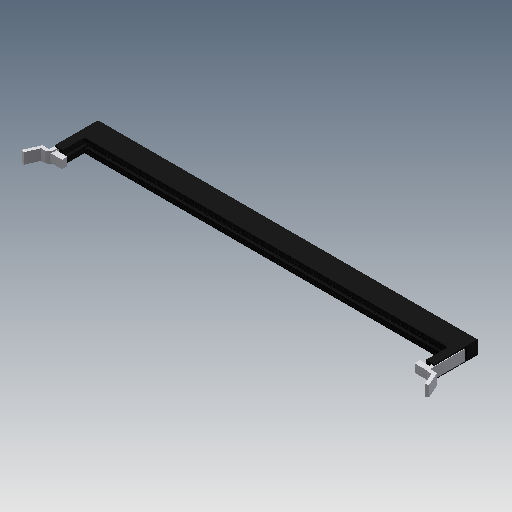
# Autodesk Inventor part: config - ram slot
Saved by Autodesk Inventor 2019.1 (Build 231200000, 200)
## iProperties
Company: Autodesk Asia Pte. Ltd.
Created: 2005-11-27
Part Number: config - ram slot
Document SubType Name: Modeling
Designer: Simon.Ng@autodesk.com
Stock Number: config - ram slot
Density: 1 g/cm^3
Material: Generic
Mass: 5.26159 g
Surface Area: 74.6749 cm^2
Volume: 5.26159 cm^3
Appearance: Glossy - Black
Title: PC Demo
Author: Simon.Ng@autodesk.com
Autodesk Inventor part; units mm, degrees
ref_plane "YZ Plane" through (0, 0, 0) normal (1, 0, 0) x (0, 1, 0)
ref_plane "XZ Plane" through (0, 0, 0) normal (0, 1, 0) x (-1, 0, 0)
ref_plane "XY Plane" through (0, 0, 0) normal (0, 0, 1) x (1, 0, 0)
sketch "Sketch1" plane through (0, 0, 0) normal (0, 0, 1) x (1, 0, 0)
  line L0 (0, 6.5) -> (0, -0.5) projected
  line L1 (-14, 0) -> (182, 0) projected
  line L2 (0, 0) -> (140, 0)
  line L3 (140, 0) -> (140, 5)
  line L4 (140, 5) -> (0, 5)
  line L5 (0, 5) -> (0, 0)
  dimension "d0" = 140
  dimension "d1" = 5
  constraints: 8 end point, 2 parallel, 2 point on line, 1 horizontal, 1 perpendicular
  measures "d0" distance of L3.end L4.end
  measures "d1" distance of L2.end L3.end
extrude "Extrusion1" add sketch "Sketch1" along normal blind 16
sketch "Sketch2" plane through (0, 0, 16) normal (0, 0, 1) x (1, 0, 0)
  line L0 (0, 0) -> (0, 5) projected
  line L1 (140, 5) -> (140, 0) projected
  line L2 (0, 2.5) -> (140, 2.5) construction
  line L3 (0, 4.5) -> (1.5, 4.5)
  line L4 (1.5, 4.5) -> (1.5, 0.5)
  line L5 (1.5, 0.5) -> (0, 0.5)
  line L6 (0, 0.5) -> (0, 4.5)
  line L7 (140, 4.5) -> (138.5, 4.5)
  line L8 (138.5, 4.5) -> (138.5, 0.5)
  line L9 (138.5, 0.5) -> (140, 0.5)
  line L10 (140, 0.5) -> (140, 4.5)
  line L11 (1.8, 3) -> (3, 3)
  line L12 (3, 3) -> (3, 2)
  line L13 (3, 2) -> (1.8, 2)
  line L14 (1.8, 2) -> (1.8, 3)
  line L15 (138.2, 3) -> (137, 3)
  line L16 (137, 3) -> (137, 2)
  line L17 (137, 2) -> (138.2, 2)
  line L18 (138.2, 2) -> (138.2, 3)
  dimension "d4" = 4
  dimension "d5" = 1.5
  dimension "d6" = 0.3
  dimension "d7" = 1.2
  dimension "d8" = 1
  dimension "d9" = 0.3
  constraints: 34 end point, 8 parallel, 4 equal length, 4 horizontal, 4 perpendicular, 2 midpoint, 2 point on line, 4 other
  measures "d4" distance of L3.end L4.end
  measures "d5" distance of L3.start L3.end
  measures "d6" distance between parallel lines of L4 L14
  measures "d7" distance of L12.end L13.end
  measures "d8" distance of L11.end L12.end
  measures "d9" distance between parallel lines of L8 L18
extrude "Extrusion2" cut sketch "Sketch2" against normal blind 12 contours L0 L3 L4 L5 | L1 L9 L8 L7
extrude "Extrusion3" cut sketch "Sketch2" against normal blind 10 contours L11 L12 L13 L14 | L18 L17 L16 L15
sketch "Sketch3" plane through (0, 0, 16) normal (0, 0, 1) x (1, 0, 0)
  line L0 (3, 3) -> (3, 2) projected
  line L1 (137, 2) -> (137, 3) projected
  line L2 (140, 0) -> (0, 0) projected
  line L3 (0, 5) -> (140, 5) projected
  line L4 (3, 5) -> (137, 5)
  line L5 (137, 5) -> (137, 0)
  line L6 (137, 0) -> (3, 0)
  line L7 (3, 0) -> (3, 5)
  constraints: 8 end point, 2 collinear, 2 parallel, 2 point on line, 1 horizontal, 1 perpendicular
extrude "Extrusion4" cut sketch "Sketch3" against normal blind 8
sketch "Sketch4" plane through (0, 0, 8) normal (0, 0, 1) x (1, 0, 0)
  line L0 (3, 5) -> (3, 3) projected
  line L1 (3, 2) -> (3, 3) projected
  line L2 (137, 3) -> (137, 2) projected
  line L3 (137, 3) -> (137, 5) projected
  line L4 (3, 2.5) -> (137, 2.5) construction
  line L5 (3, 3.5) -> (4, 3.5)
  line L6 (4, 3.5) -> (4, 1.5)
  line L7 (4, 1.5) -> (3, 1.5)
  line L8 (3, 1.5) -> (3, 3.5)
  line L9 (137, 3.7646) -> (136, 3.7646)
  line L10 (136, 3.7646) -> (136, 1.2354)
  line L11 (136, 1.2354) -> (137, 1.2354)
  line L12 (137, 1.2354) -> (137, 3.7646)
  dimension "d16" = 1
  dimension "d17" = 2
  constraints: 18 end point, 5 parallel, 2 horizontal, 2 midpoint, 2 perpendicular, 2 point on line, 2 other
  measures "d16" distance of L5.start L5.end
  measures "d17" distance of L5.end L6.end
extrude "Extrusion5" cut sketch "Sketch4" against normal up to surface (2 mm away)
sketch "Sketch5" plane through (138.2, 2, 6) normal (-1, 0, 0) x (0, 0, 1)
  line L0 (0, 0) -> (0, 1) projected
  line L1 (10, 0) -> (0, 0) projected
  line L2 (10, 1) -> (10, 0) projected
  line L3 (10, 1) -> (0, 1) projected
  line L4 (7, 1) -> (7, 0)
  dimension "d20" = 3
  constraints: 2 end point, 2 point on line, 1 parallel, 1 perpendicular
  measures "d20" distance between parallel lines of L2 L4
extrude "Extrusion6" cut sketch "Sketch5" against normal through all contours L0 L3 L4 L1
ref_plane "Work Plane1" through (70, 0, 0) normal (-1, 0, 0) x (0, 0, 1)
mirror "Mirror1" about plane through (70, 0, 0) normal (-1, 0, 0) of "Extrusion6"
sketch "Sketch6" plane through (0, 0, 8) normal (0, 0, 1) x (1, 0, 0)
  line L0 (4, 3.5) -> (4, 1.5) projected
  line L1 (136, 1.2354) -> (136, 3.7646) projected
  line L2 (4, 2.5) -> (136, 2.5) construction
  line L3 (4, 3) -> (136, 3)
  line L4 (136, 3) -> (136, 2)
  line L5 (136, 2) -> (4, 2)
  line L6 (4, 2) -> (4, 3)
  dimension "d23" = 1
  constraints: 10 end point, 2 midpoint, 2 parallel, 2 point on line, 1 horizontal, 1 perpendicular, 1 other
  measures "d23" distance between parallel lines of L5 L3
extrude "Extrusion7" cut sketch "Sketch6" against normal blind 3
sketch "Sketch7" plane through (0, 0, 8) normal (0, 0, 1) x (1, 0, 0)
  line L0 (4, 3) -> (136, 3) projected
  line L1 (3, 5) -> (137, 5) projected
  line L2 (136, 2) -> (4, 2) projected
  line L3 (4, 2) -> (4, 1.5) projected
  line L4 (4, 1.5) -> (3, 1.5) projected
  line L5 (3, 1.5) -> (3, 0) projected
  line L6 (137, 0) -> (3, 0) projected
  line L7 (137, 0) -> (137, 1.2354) projected
  line L8 (137, 1.2354) -> (136, 1.2354) projected
  line L9 (136, 1.2354) -> (136, 2) projected
  line L10 (8.6043, 5) -> (8.6043, 3) construction
  line L11 (8.6043, 2) -> (8.6043, 0) construction
  line L12 (8.6043, 4) -> (7.6918, 4) construction
  line L13 (8.6043, 1) -> (8.0236, 1) construction
  line L14 (4.375, 4.6) -> (4.625, 4.6)
  line L15 (4.625, 4.6) -> (4.625, 3.4)
  line L16 (4.625, 3.4) -> (4.375, 3.4)
  line L17 (4.375, 3.4) -> (4.375, 4.6)
  line L18 (4.375, 1.6) -> (4.625, 1.6)
  line L19 (4.625, 1.6) -> (4.625, 0.4)
  line L20 (4.625, 0.4) -> (4.375, 0.4)
  line L21 (4.375, 0.4) -> (4.375, 1.6)
  line L22 (4, 3.5) -> (4, 3) projected
  dimension "d26" = 1.2
  dimension "d28" = 0.25
  dimension "d37" = 0.375
  constraints: 24 end point, 5 parallel, 4 collinear, 4 perpendicular, 4 point on line, 2 horizontal, 2 midpoint, 2 other
  measures "d26" distance of L14.end L15.end
  measures "d28" distance of L14.start L14.end
  measures "d37" distance between parallel lines of L22 L17
extrude "Extrusion8" cut sketch "Sketch7" against normal blind 2.5 contours L14 L15 L16 L17 | L18 L19 L20 L21
sketch "Sketch8" plane through (4.375, 1.6, 5.5) normal (0, -1, 0) x (1, 0, 0)
  line L0 (0.25, 0) -> (0, 0) projected
  line L1 (0.25, 2.5) -> (0.25, 0) projected
  line L2 (0, 2.5) -> (0.25, 2.5) projected
  line L3 (0, 2.5) -> (0, 0) projected
  line L4 (0, 2) -> (0.25, 2)
  dimension "d31" = 0.5
  constraints: 2 end point, 2 point on line, 1 perpendicular
  measures "d31" distance between parallel lines of L4 L2
extrude "Extrusion9" cut sketch "Sketch8" against normal up to surface (1.8 mm away) contours L0 L3 L4 L1
pattern_linear "Rectangular Pattern1" count 132 spacing 1 along (1, 0, 0) of "Extrusion9", "Extrusion8"
sketch "Sketch9" plane through (0, 0.5, 4) normal (0, 1, 0) x (-1, 0, 0)
  line L0 (0, 0) -> (-1.5, 0) projected
  line L1 (0, 12) -> (0, 0) projected
  line L2 (-1.5, 12) -> (-1.5, 0) projected
  line L3 (-1, 1) -> (-1, 13)
  arc A0 (0.5, 14.9365) -> (-1, 13) centre (1, 13) ccw
  line L4 (0.5, 14.9365) -> (2, 14.9365)
  line L5 (2, 14.9365) -> (4, 19.4365)
  line L6 (5.0966, 18.9491) -> (2.7798, 13.7365)
  line L7 (2.7798, 13.7365) -> (0.6876, 13.7365)
  arc A1 (0.6876, 13.7365) -> (0.2, 13) centre (1, 13) ccw
  line L8 (0.2, 13) -> (0.2, 1)
  line L9 (5.0966, 18.9491) -> (4, 19.4365)
  line L10 (0.2, 1) -> (-1, 1)
  dimension "d38" = 12
  dimension "d39" = 2
  dimension "d40" = 1.5
  dimension "d41" = 0.5
  dimension "d42" = 1
  dimension "d43" = 4.5
  dimension "d44" = 3
  dimension "d45" = 2
  dimension "d46" = 1.2
  constraints: 16 end point, 4 perpendicular, 4 point on circle, 2 centre point, 2 parallel, 1 tangent, 3 other
  measures "d38" distance of L3.start L3.end
  measures "d39" radius of A0
  measures "d40" distance of L4.start L4.end
  measures "d41" distance between parallel lines of L2 L3
  measures "d42" distance from line of L0 L3.start
  measures "d43" vertical distance of L4.end L5.end
  measures "d44" distance from line of L3 L4.end
  measures "d45" horizontal distance of L4.end L5.end
  measures "d46" distance between parallel lines of L3 L8
extrude "Extrusion10" add sketch "Sketch9" along normal up to surface (4 mm away)
ref_plane "Work Plane3" through (5, 0.5, 17) normal (1, 0, 0) x (0, 0, -1)
sketch "Sketch10" plane through (5, 0.5, 17) normal (1, 0, 0) x (0, 0, -1)
  line L0 (0, 0) -> (0, 4) construction
  line L1 (0, 2) -> (-3.348, 2) construction
  line L2 (-1.25, 3.5) -> (0.75, 3.5)
  line L3 (0.75, 3.5) -> (0.75, 0.5)
  line L4 (0.75, 0.5) -> (-1.25, 0.5)
  line L5 (-1.25, 0.5) -> (-1.25, 3.5)
  line L6 (1, 0) -> (1, 4) projected
  dimension "d51" = 3
  dimension "d52" = 2
  dimension "d55" = 0.25
  constraints: 10 end point, 2 parallel, 2 perpendicular, 1 horizontal, 1 midpoint, 1 other
  measures "d51" distance of L4.end L2.start
  measures "d52" distance of L2.start L2.end
  measures "d55" distance between parallel lines of L6 L3
extrude "Extrusion11" add sketch "Sketch10" against normal up to next
ref_plane "Work Plane4" through (70, 0, 0) normal (-1, 0, 0) x (0, 0, 1)
mirror "Mirror2" about plane through (70, 0, 0) normal (-1, 0, 0) of "Extrusion11", "Extrusion10"
equation "\"d9\" = d6"
body "Solid1"
